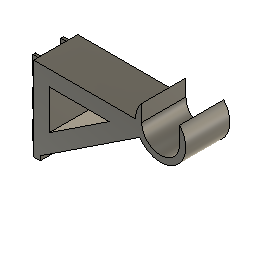
spool_rod_bracket (Autodesk Fusion 360 design; units mm, degrees)
part number: 2026-09-02-15-09-45-457
Autodesk Fusion 360 part; units mm, degrees
sketch "Arm triangle" plane through (0, 0, 0) normal (0, 1, 0) x (1, 0, 0)
  line L0 (0, 0) -> (0, -76)
  line L1 (0, -76) -> (115, -76)
  line L2 (115, -76) -> (0, 0)
extrude "Arm triangle (1)" add sketch "Arm triangle" along normal mid plane 40
sketch "Hook plate" plane through (0, 0, 0) normal (0, 1, 0) x (1, 0, 0)
  line L0 (0, 0) -> (6, 0)
  line L1 (6, 0) -> (6, -76)
  line L2 (6, -76) -> (0, -76)
  line L3 (0, -76) -> (0, 0)
extrude "Hook plate (1)" add sketch "Hook plate" along normal mid plane 40
sketch "Saddle boss" plane through (0, 0, 0) normal (0, 1, 0) x (1, 0, 0)
  circle A0 centre (115, -76) radius 22.7
extrude "Saddle boss (1)" add sketch "Saddle boss" along normal mid plane 40
sketch "Lightening cutout" plane through (0, 0, 0) normal (0, 1, 0) x (1, 0, 0)
  line L0 (14, -26.0332) -> (14, -62)
  line L1 (14, -62) -> (68.4235, -62)
  line L2 (68.4235, -62) -> (14, -26.0332)
extrude "Lightening cutout (1)" cut sketch "Lightening cutout" along normal mid plane 50
sketch "Rod pocket" plane through (0, 0, 0) normal (0, 1, 0) x (1, 0, 0)
  circle A0 centre (115, -76) radius 17.1
extrude "Rod pocket (1)" cut sketch "Rod pocket" along normal mid plane 50
sketch "Rod drop-in opening" plane through (0, 0, 0) normal (0, 1, 0) x (1, 0, 0)
  line L0 (97.9, -76) -> (132.1, -76)
  line L1 (132.1, -76) -> (132.1, -103.7)
  line L2 (132.1, -103.7) -> (97.9, -103.7)
  line L3 (97.9, -103.7) -> (97.9, -76)
extrude "Rod drop-in opening (1)" cut sketch "Rod drop-in opening" along normal mid plane 50
sketch "Hook profiles" plane through (0, 0, 0) normal (0, 1, 0) x (1, 0, 0)
  line L0 (0, -74) -> (-6.8, -74)
  line L1 (-6.8, -74) -> (-6.8, -57)
  line L2 (-6.8, -57) -> (-2.8, -57)
  line L3 (-2.8, -57) -> (-2.8, -69)
  line L4 (-2.8, -69) -> (0, -69)
  line L5 (0, -69) -> (0, -74)
  line L6 (0, -48.6) -> (-6.8, -48.6)
  line L7 (-6.8, -48.6) -> (-6.8, -31.6)
  line L8 (-6.8, -31.6) -> (-2.8, -31.6)
  line L9 (-2.8, -31.6) -> (-2.8, -43.6)
  line L10 (-2.8, -43.6) -> (0, -43.6)
  line L11 (0, -43.6) -> (0, -48.6)
  line L12 (0, -23.2) -> (-6.8, -23.2)
  line L13 (-6.8, -23.2) -> (-6.8, -6.2)
  line L14 (-6.8, -6.2) -> (-2.8, -6.2)
  line L15 (-2.8, -6.2) -> (-2.8, -18.2)
  line L16 (-2.8, -18.2) -> (0, -18.2)
  line L17 (0, -18.2) -> (0, -23.2)
extrude "Hook slab" add sketch "Hook profiles" along normal mid plane 27.8
extrude "Hook column split" cut sketch "Hook profiles" along normal mid plane 23
named bodies: "spool_rod_bracket"
